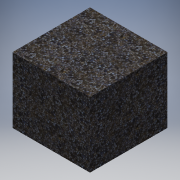
# Autodesk Inventor part: 2p3cem
Saved by Autodesk Inventor 2016 (Build 200138000, 138)
## iProperties
Company: HERA Project
Created: 2013-06-11
Part Number: 2p3cem
Material: Concrete
Document SubType Name: Modeling
Designer: David DeBoer
Density: 2.40731 g/cm^3
Description: Support stand cement
Mass: 39212.8 g
Surface Area: 3562.79 cm^2
Volume: 16289.1 cm^3
Appearance: Exposed Aggregate - Coarse
Author: David DeBoer
Title: Support stand cement
Autodesk Inventor part; units mm, degrees
ref_plane "YZ Plane" through (0, 0, 0) normal (1, 0, 0) x (0, 1, 0)
ref_plane "XZ Plane" through (0, 0, 0) normal (0, 1, 0) x (-1, 0, 0)
ref_plane "XY Plane" through (0, 0, 0) normal (0, 0, 1) x (1, 0, 0)
sketch "Sketch1" plane through (0, 0, 0) normal (0, 1, 0) x (-1, 0, 0)
  line L0 (150, 150) -> (150, -150)
  line L1 (150, -150) -> (-150, -150)
  line L2 (-150, -150) -> (-150, 150)
  line L3 (-150, 150) -> (150, 150)
  point P0 (0, 0)
  dimension "d5" = 150
  dimension "d6" = 150
  dimension "d7" = 300
  dimension "d8" = 300
  dimension "d9" = 300
  constraints: 8 end point, 1 horizontal, 1 perpendicular, 1 vertical
  measures "d5" distance from line of point (0, 0) L0
  measures "d6" horizontal distance of L0.start point (0, 0)
  measures "d7" distance of L0.start L0.end
  measures "d8" distance of L0.end L1.end
  measures "d9" distance of L1.end L2.end
extrude "Extrusion1" add sketch "Sketch1" against normal blind 254
sketch "Sketch2" plane through (0, -254, 0) normal (0, -1, 0) x (1, 0, 0)
  circle A0 centre (0, 0) radius 15
  dimension "d10" = 30
  constraints: 1 centre point, 1 coincident
  measures "d10" diameter of A0
extrude "Extrusion2" add sketch "Sketch2" against normal blind 10 separate body
body "Solid1"
body "Solid2"
